Autodesk Fusion 360 part; units mm, degrees
(part 15 of 25)
  arc A3929 (0.7747, 17.3038) -> (0.7747, 16.9862) centre (0.7747, 17.145) ccw
  arc A3930 (40.64, 16.6688) -> (40.64, 16.3513) centre (40.64, 16.51) ccw
  arc A3931 (45.607, 16.3513) -> (45.607, 16.6688) centre (45.607, 16.51) ccw
  arc A3932 (16.0714, 16.6688) -> (16.0714, 16.3513) centre (16.0714, 16.51) ccw
  arc A3933 (44.7421, 18.8912) -> (44.7421, 19.2088) centre (44.7421, 19.05) ccw
  arc A3934 (53.34, 16.3513) -> (53.34, 16.6688) centre (53.34, 16.51) ccw
  arc A3935 (44.972, 16.9862) -> (44.972, 17.3038) centre (44.972, 17.145) ccw
  arc A3936 (68.404, 17.3038) -> (68.404, 16.9862) centre (68.404, 17.145) ccw
  arc A3937 (53.34, 17.9388) -> (53.34, 17.6212) centre (53.34, 17.78) ccw
  arc A3938 (49.2073, 16.9862) -> (49.2073, 17.3038) centre (49.2073, 17.145) ccw
  arc A3939 (24.1735, 17.6212) -> (24.1735, 17.9388) centre (24.1735, 17.78) ccw
  arc A3940 (26.7135, 17.6212) -> (26.7135, 17.9388) centre (26.7135, 17.78) ccw
  arc A3941 (29.2535, 17.6212) -> (29.2535, 17.9388) centre (29.2535, 17.78) ccw
  arc A3942 (57.898, 18.5738) -> (57.898, 18.2562) centre (57.898, 18.415) ccw
  arc A3943 (73.5304, 18.2562) -> (73.5304, 18.5738) centre (73.5304, 18.415) ccw
  arc A3944 (68.2336, 17.6212) -> (68.2336, 17.9388) centre (68.2336, 17.78) ccw
  arc A3945 (49.6453, 16.3513) -> (49.6453, 16.6688) centre (49.6453, 16.51) ccw
  arc A3946 (84.2253, 16.9862) -> (84.2253, 17.3038) centre (84.2253, 17.145) ccw
  arc A3947 (70.8314, 18.5738) -> (70.8314, 18.2562) centre (70.8314, 18.415) ccw
  arc A3948 (46.6979, 19.2088) -> (46.6979, 18.8912) centre (46.6979, 19.05) ccw
  arc A3949 (53.34, 16.6688) -> (53.34, 16.3513) centre (53.34, 16.51) ccw
  arc A3950 (54.7705, 17.3038) -> (54.7705, 16.9862) centre (54.7705, 17.145) ccw
  arc A3951 (34.2465, 17.9388) -> (34.2465, 17.6212) centre (34.2465, 17.78) ccw
  arc A3952 (40.64, 16.9862) -> (40.64, 17.3038) centre (40.64, 17.145) ccw
  arc A3953 (56.402, 16.9862) -> (56.402, 17.3038) centre (56.402, 17.145) ccw
  arc A3954 (54.1355, 16.6688) -> (54.1355, 16.3513) centre (54.1355, 16.51) ccw
  arc A3955 (24.0865, 17.9388) -> (24.0865, 17.6212) centre (24.0865, 17.78) ccw
  arc A3956 (40.64, 17.3038) -> (40.64, 16.9862) centre (40.64, 17.145) ccw
  arc A3957 (80.0328, 18.2562) -> (80.0328, 18.5738) centre (80.0328, 18.415) ccw
  arc A3958 (0.7747, 19.2088) -> (0.7747, 18.8912) centre (0.7747, 19.05) ccw
  arc A3959 (51.9547, 19.2088) -> (51.9547, 18.8912) centre (51.9547, 19.05) ccw
  arc A3960 (55.767, 17.6212) -> (55.767, 17.9388) centre (55.767, 17.78) ccw
  line L1372 (57.263, 19.05) -> (57.5886, 19.05)
  arc A3961 (81.5721, 18.2562) -> (81.5721, 18.5738) centre (81.5721, 18.415) ccw
  arc A3962 (36.7865, 17.9388) -> (36.7865, 17.6212) centre (36.7865, 17.78) ccw
  arc A3963 (54.1355, 19.2088) -> (54.1355, 18.8912) centre (54.1355, 19.05) ccw
  arc A3964 (0.7747, 18.5738) -> (0.7747, 18.2562) centre (0.7747, 18.415) ccw
  arc A3965 (40.64, 17.6212) -> (40.64, 17.9388) centre (40.64, 17.78) ccw
  arc A3966 (83.5279, 19.8438) -> (83.5279, 19.5263) centre (83.5279, 19.6851) ccw
  arc A3967 (84.2253, 19.5263) -> (84.2253, 19.8438) centre (84.2253, 19.6851) ccw
  arc A3968 (40.64, 17.9388) -> (40.64, 17.6212) centre (40.64, 17.78) ccw
  line L1373 (39.3265, 17.78) -> (39.8168, 17.78)
  arc A3969 (56.9341, 20.1612) -> (56.9341, 20.4788) centre (56.9341, 20.32) ccw
  arc A3970 (70.1964, 20.4788) -> (70.1964, 20.1612) centre (70.1964, 20.32) ccw
  arc A3971 (44.7421, 20.1612) -> (44.7421, 20.4788) centre (44.7421, 20.32) ccw
  arc A3972 (6.2857, 20.1612) -> (6.2857, 20.4788) centre (6.2857, 20.32) ccw
  arc A3973 (36.8735, 17.6212) -> (36.8735, 17.9388) centre (36.8735, 17.78) ccw
  arc A3974 (83.5279, 18.5738) -> (83.5279, 18.2562) centre (83.5279, 18.415) ccw
  arc A3975 (44.7421, 18.2562) -> (44.7421, 18.5738) centre (44.7421, 18.415) ccw
  arc A3976 (41.4632, 17.9388) -> (41.4632, 17.6212) centre (41.4632, 17.78) ccw
  arc A3977 (79.2208, 20.1612) -> (79.2208, 20.4788) centre (79.2208, 20.32) ccw
  line L1374 (81.4096, 18.415) -> (81.5721, 18.415)
  arc A3978 (53.34, 18.5738) -> (53.34, 18.2562) centre (53.34, 18.415) ccw
  arc A3979 (72.7184, 20.1612) -> (72.7184, 20.4788) centre (72.7184, 20.32) ccw
  arc A3980 (84.2253, 20.1612) -> (84.2253, 20.4788) centre (84.2253, 20.32) ccw
  arc A3981 (8.9543, 20.4788) -> (8.9543, 20.1612) centre (8.9543, 20.32) ccw
  arc A3982 (46.6979, 18.5738) -> (46.6979, 18.2562) centre (46.6979, 18.415) ccw
  arc A3983 (75.7192, 20.4788) -> (75.7192, 20.1612) centre (75.7192, 20.32) ccw
  arc A3984 (59.2514, 19.2088) -> (59.2514, 18.8912) centre (59.2514, 19.05) ccw
  arc A3985 (83.3742, 20.4788) -> (83.3742, 20.1612) centre (83.3742, 20.32) ccw
  line L1375 (36.7865, 17.78) -> (36.8735, 17.78)
  arc A3986 (7.62, 20.1612) -> (7.62, 20.4788) centre (7.62, 20.32) ccw
  arc A3987 (39.8168, 17.6212) -> (39.8168, 17.9388) centre (39.8168, 17.78) ccw
  line L1376 (54.7705, 18.415) -> (55.132, 18.415)
  arc A3988 (53.34, 18.2562) -> (53.34, 18.5738) centre (53.34, 18.415) ccw
  arc A3989 (81.4096, 18.5738) -> (81.4096, 18.2562) centre (81.4096, 18.415) ccw
  arc A3990 (74.9072, 18.5738) -> (74.9072, 18.2562) centre (74.9072, 18.415) ccw
  arc A3991 (53.34, 19.2088) -> (53.34, 18.8912) centre (53.34, 19.05) ccw
  arc A3992 (44.7421, 17.6212) -> (44.7421, 17.9388) centre (44.7421, 17.78) ccw
  arc A3993 (47.103, 17.9388) -> (47.103, 17.6212) centre (47.103, 17.78) ccw
  arc A3994 (84.2253, 17.6212) -> (84.2253, 17.9388) centre (84.2253, 17.78) ccw
  arc A3995 (49.2073, 18.2562) -> (49.2073, 18.5738) centre (49.2073, 18.415) ccw
  arc A3996 (53.34, 18.8912) -> (53.34, 19.2088) centre (53.34, 19.05) ccw
  arc A3997 (49.0855, 17.6212) -> (49.0855, 17.9388) centre (49.0855, 17.78) ccw
  arc A3998 (54.9021, 18.8912) -> (54.9021, 19.2088) centre (54.9021, 19.05) ccw
  arc A3999 (58.533, 17.9388) -> (58.533, 17.6212) centre (58.533, 17.78) ccw
  arc A4000 (55.132, 18.2562) -> (55.132, 18.5738) centre (55.132, 18.415) ccw
  arc A4001 (67.6058, 18.2562) -> (67.6058, 18.5738) centre (67.6058, 18.415) ccw
  arc A4002 (84.2253, 18.2562) -> (84.2253, 18.5738) centre (84.2253, 18.415) ccw
  arc A4003 (0.7747, 21.1138) -> (0.7747, 20.7963) centre (0.7747, 20.955) ccw
  arc A4004 (7.62, 21.1138) -> (7.62, 20.7963) centre (7.62, 20.955) ccw
  arc A4005 (56.9536, 19.5263) -> (56.9536, 19.8438) centre (56.9536, 19.6851) ccw
  arc A4006 (7.62, 20.4788) -> (7.62, 20.1612) centre (7.62, 20.32) ccw
  arc A4007 (57.5886, 18.8912) -> (57.5886, 19.2088) centre (57.5886, 19.05) ccw
  arc A4008 (57.263, 19.2088) -> (57.263, 18.8912) centre (57.263, 19.05) ccw
  arc A4009 (83.5279, 19.2088) -> (83.5279, 18.8912) centre (83.5279, 19.05) ccw
  arc A4010 (5.7785, 20.7963) -> (5.7785, 21.1138) centre (5.7785, 20.955) ccw
  arc A4011 (7.62, 20.7963) -> (7.62, 21.1138) centre (7.62, 20.955) ccw
  arc A4012 (84.2253, 18.8912) -> (84.2253, 19.2088) centre (84.2253, 19.05) ccw
  arc A4013 (74.9072, 19.8438) -> (74.9072, 19.5263) centre (74.9072, 19.6851) ccw
  arc A4014 (0.7747, 19.8438) -> (0.7747, 19.5263) centre (0.7747, 19.6851) ccw
  arc A4015 (46.6979, 20.4788) -> (46.6979, 20.1612) centre (46.6979, 20.32) ccw
  line L1377 (56.8579, 20.32) -> (56.9341, 20.32)
  arc A4016 (56.8579, 20.4788) -> (56.8579, 20.1612) centre (56.8579, 20.32) ccw
  arc A4017 (67.0941, 20.1612) -> (67.0941, 20.4788) centre (67.0941, 20.32) ccw
  arc A4018 (59.9059, 20.4788) -> (59.9059, 20.1612) centre (59.9059, 20.32) ccw
  arc A4019 (0.7747, 20.4788) -> (0.7747, 20.1612) centre (0.7747, 20.32) ccw
  arc A4020 (46.6979, 19.8438) -> (46.6979, 19.5263) centre (46.6979, 19.6851) ccw
  arc A4021 (54.9021, 19.5263) -> (54.9021, 19.8438) centre (54.9021, 19.6851) ccw
  arc A4022 (71.4591, 21.7488) -> (71.4591, 21.4312) centre (71.4591, 21.59) ccw
  arc A4023 (84.2253, 21.4312) -> (84.2253, 21.7488) centre (84.2253, 21.59) ccw
  arc A4024 (44.7421, 19.5263) -> (44.7421, 19.8438) centre (44.7421, 19.6851) ccw
  arc A4025 (81.5721, 18.8912) -> (81.5721, 19.2088) centre (81.5721, 19.05) ccw
  arc A4026 (7.62, 22.0663) -> (7.62, 22.3838) centre (7.62, 22.2251) ccw
  arc A4027 (7.62, 22.3838) -> (7.62, 22.0663) centre (7.62, 22.2251) ccw
  arc A4028 (56.8579, 21.7488) -> (56.8579, 21.4312) centre (56.8579, 21.59) ccw
  line L1378 (56.8579, 19.685) -> (56.9536, 19.685)
  line L1379 (56.8579, 20.955) -> (56.9536, 20.955)
  arc A4029 (56.8579, 19.8438) -> (56.8579, 19.5263) centre (56.8579, 19.6851) ccw
  arc A4030 (44.464, 20.7963) -> (44.464, 21.1138) centre (44.464, 20.955) ccw
  arc A4031 (43.194, 22.0663) -> (43.194, 22.3838) centre (43.194, 22.2251) ccw
  arc A4032 (70.0464, 19.8438) -> (70.0464, 19.5263) centre (70.0464, 19.6851) ccw
  arc A4033 (70.1964, 19.2088) -> (70.1964, 18.8912) centre (70.1964, 19.05) ccw
  arc A4034 (67.437, 18.8912) -> (67.437, 19.2088) centre (67.437, 19.05) ccw
  arc A4035 (54.9021, 20.1612) -> (54.9021, 20.4788) centre (54.9021, 20.32) ccw
  arc A4036 (59.8864, 19.8438) -> (59.8864, 19.5263) centre (59.8864, 19.6851) ccw
  arc A4037 (80.0328, 19.5263) -> (80.0328, 19.8438) centre (80.0328, 19.6851) ccw
  arc A4038 (59.2514, 21.7488) -> (59.2514, 21.4312) centre (59.2514, 21.59) ccw
  arc A4039 (73.5304, 19.5263) -> (73.5304, 19.8438) centre (73.5304, 19.6851) ccw
  arc A4040 (72.4535, 21.4312) -> (72.4535, 21.7488) centre (72.4535, 21.59) ccw
  arc A4041 (67.1136, 19.5263) -> (67.1136, 19.8438) centre (67.1136, 19.6851) ccw
  arc A4042 (5.7785, 22.0663) -> (5.7785, 22.3838) centre (5.7785, 22.2251) ccw
  arc A4043 (48.9268, 17.439) -> (49.2443, 17.439) centre (49.0856, 17.439) ccw
  line L1380 (53.34, 17.78) -> (53.34, 16.3195)
  line L1381 (51.7712, 16.3265) -> (52.2496, 16.8049)
  arc A4044 (54.6417, 17.175) -> (54.9592, 17.175) centre (54.8005, 17.175) ccw
  arc A4045 (57.5886, 21.4312) -> (57.5886, 21.7488) centre (57.5886, 21.59) ccw
  arc A4046 (82.7392, 21.1138) -> (82.7392, 20.7963) centre (82.7392, 20.955) ccw
  arc A4047 (53.1813, 17.78) -> (53.4988, 17.78) centre (53.3401, 17.78) ccw
  arc A4048 (45.96, 22.3838) -> (45.96, 22.0663) centre (45.96, 22.2251) ccw
  arc A4049 (54.9021, 22.0663) -> (54.9021, 22.3838) centre (54.9021, 22.2251) ccw
  arc A4050 (53.34, 17.9387) -> (53.34, 17.6212) centre (53.34, 17.78) ccw
  arc A4051 (54.9021, 20.7963) -> (54.9021, 21.1138) centre (54.9021, 20.955) ccw
  arc A4052 (48.9388, 18.1818) -> (49.2322, 18.0603) centre (49.0855, 18.1211) ccw
  line L1382 (54.8005, 17.175) -> (54.8005, 17.78)
  arc A4053 (53.4987, 17.78) -> (53.1812, 17.78) centre (53.34, 17.78) ccw
  arc A4054 (56.8579, 21.1138) -> (56.8579, 20.7963) centre (56.8579, 20.955) ccw
  arc A4055 (72.4553, 20.7963) -> (72.4553, 21.1138) centre (72.4553, 20.955) ccw
  arc A4056 (54.9592, 18.385) -> (54.6417, 18.385) centre (54.8005, 18.385) ccw
  line L1383 (54.8005, 18.385) -> (53.945, 19.2405)
  line L1384 (49.8288, 19.2335) -> (49.3465, 18.7512)
  arc A4057 (0.7747, 22.3838) -> (0.7747, 22.0663) centre (0.7747, 22.2251) ccw
  line L1385 (54.8005, 17.78) -> (53.34, 17.78)
  line L1386 (54.8005, 17.78) -> (54.8005, 18.385)
  arc A4058 (51.6589, 16.4388) -> (51.8834, 16.2143) centre (51.7712, 16.3266) ccw
  line L1387 (53.34, 16.3195) -> (53.945, 16.3195)
  arc A4059 (46.6979, 21.1138) -> (46.6979, 20.7963) centre (46.6979, 20.955) ccw
  arc A4060 (53.1813, 16.3195) -> (53.4988, 16.3195) centre (53.3401, 16.3195) ccw
  arc A4061 (51.141, 15.9068) -> (51.141, 16.2243) centre (51.141, 16.0655) ccw
  line L1388 (52.2496, 16.8049) -> (52.735, 16.3195)
  arc A4062 (53.945, 16.1608) -> (53.945, 16.4783) centre (53.945, 16.3195) ccw
  arc A4063 (82.663, 21.7488) -> (82.663, 21.4312) centre (82.663, 21.59) ccw
  arc A4064 (7.62, 21.7488) -> (7.62, 21.4312) centre (7.62, 21.59) ccw
  arc A4065 (54.9021, 21.4312) -> (54.9021, 21.7488) centre (54.9021, 21.59) ccw
  arc A4066 (67.1136, 20.7963) -> (67.1136, 21.1138) centre (67.1136, 20.955) ccw
  arc A4067 (56.9536, 20.7963) -> (56.9536, 21.1138) centre (56.9536, 20.955) ccw
  arc A4068 (54.0572, 19.3528) -> (53.8327, 19.1282) centre (53.945, 19.2405) ccw
  arc A4069 (70.8314, 21.1138) -> (70.8314, 20.7963) centre (70.8314, 20.955) ccw
  line L1389 (53.945, 19.2405) -> (53.34, 19.2405)
  arc A4070 (67.7486, 21.4312) -> (67.7486, 21.7488) centre (67.7486, 21.59) ccw
  arc A4071 (52.6228, 16.2072) -> (52.8473, 16.4318) centre (52.7351, 16.3195) ccw
  arc A4072 (54.8005, 17.6213) -> (54.8005, 17.9388) centre (54.8005, 17.78) ccw
  arc A4073 (9.4615, 22.3838) -> (9.4615, 22.0663) centre (9.4615, 22.2251) ccw
  line L1390 (53.34, 17.78) -> (54.8005, 17.78)
  arc A4074 (46.3862, 22.0233) -> (46.1617, 21.7988) centre (46.2739, 21.9111) ccw
  arc A4075 (84.2253, 20.7963) -> (84.2253, 21.1138) centre (84.2253, 20.955) ccw
  arc A4076 (9.4615, 21.1138) -> (9.4615, 20.7963) centre (9.4615, 20.955) ccw
  arc A4077 (0.7747, 21.7488) -> (0.7747, 21.4312) centre (0.7747, 21.59) ccw
  arc A4078 (43.829, 21.4312) -> (43.829, 21.7488) centre (43.829, 21.59) ccw
  arc A4079 (46.568, 21.7488) -> (46.568, 21.4312) centre (46.568, 21.59) ccw
  arc A4080 (49.4932, 18.6904) -> (49.1998, 18.8119) centre (49.3465, 18.7512) ccw
  arc A4081 (53.34, 17.9388) -> (53.34, 17.6213) centre (53.34, 17.78) ccw
  line L1391 (46.2739, 21.911) -> (43.1258, 25.0591)
  arc A4082 (7.62, 21.4312) -> (7.62, 21.7488) centre (7.62, 21.59) ccw
  arc A4083 (59.8864, 21.1138) -> (59.8864, 20.7963) centre (59.8864, 20.955) ccw
  arc A4084 (54.6417, 17.78) -> (54.9592, 17.78) centre (54.8005, 17.78) ccw
  arc A4085 (12.1476, 33.5781) -> (12.465, 33.5781) centre (12.3063, 33.5781) ccw
  line L1392 (51.141, 16.0655) -> (51.7712, 16.3265)
  arc A4086 (49.1998, 16.7481) -> (49.4932, 16.8696) centre (49.3465, 16.8088) ccw
  arc A4087 (49.9411, 19.1212) -> (49.7166, 19.3457) centre (49.8288, 19.2335) ccw
  line L1393 (49.3465, 16.8088) -> (49.8288, 16.3265)
  arc A4088 (52.3619, 16.9172) -> (52.1374, 16.6927) centre (52.2497, 16.8049) ccw
  line L1394 (53.945, 16.3195) -> (54.8005, 17.175)
  arc A4089 (53.34, 16.4783) -> (53.34, 16.1608) centre (53.34, 16.3195) ccw
  arc A4090 (51.0803, 16.2122) -> (51.2018, 15.9188) centre (51.1411, 16.0655) ccw
  arc A4091 (50.459, 16.2243) -> (50.459, 15.9068) centre (50.459, 16.0655) ccw
  arc A4092 (53.8327, 16.4318) -> (54.0572, 16.2072) centre (53.9449, 16.3195) ccw
  arc A4093 (54.9592, 17.78) -> (54.6417, 17.78) centre (54.8005, 17.78) ccw
  arc A4094 (54.9128, 17.0628) -> (54.6882, 17.2873) centre (54.8005, 17.175) ccw
  arc A4095 (49.2443, 18.121) -> (48.9268, 18.121) centre (49.0856, 18.121) ccw
  arc A4096 (49.2343, 18.8634) -> (49.4588, 18.6389) centre (49.3465, 18.7512) ccw
  arc A4097 (53.34, 16.1608) -> (53.34, 16.4783) centre (53.34, 16.3195) ccw
  arc A4098 (52.3619, 16.6927) -> (52.1374, 16.9172) centre (52.2497, 16.805) ccw
  line L1395 (49.3465, 18.7512) -> (49.0855, 18.121)
  arc A4099 (53.34, 17.9387) -> (53.34, 17.6212) centre (53.34, 17.78) ccw
  line L1396 (52.735, 16.3195) -> (53.34, 16.3195)
  arc A4100 (49.8896, 16.4732) -> (49.7681, 16.1798) centre (49.8289, 16.3265) ccw
  arc A4101 (53.1812, 16.3195) -> (53.4987, 16.3195) centre (53.34, 16.3195) ccw
  arc A4102 (51.8319, 16.1798) -> (51.7104, 16.4732) centre (51.7712, 16.3265) ccw
  arc A4103 (53.4988, 17.78) -> (53.1813, 17.78) centre (53.3401, 17.78) ccw
  line L1397 (53.34, 16.3195) -> (53.34, 17.78)
  line L1398 (49.8288, 16.3265) -> (50.459, 16.0655)
  line L1399 (50.459, 16.0655) -> (51.141, 16.0655)
  line L1400 (49.0855, 17.439) -> (49.3465, 16.8088)
  arc A4104 (52.735, 16.4783) -> (52.735, 16.1608) centre (52.735, 16.3195) ccw
  line L1401 (49.0855, 18.121) -> (49.0855, 17.439)
  arc A4105 (50.3982, 15.9188) -> (50.5197, 16.2122) centre (50.459, 16.0655) ccw
  arc A4106 (54.8005, 17.6212) -> (54.8005, 17.9387) centre (54.8005, 17.78) ccw
  arc A4107 (53.34, 17.6212) -> (53.34, 17.9387) centre (53.34, 17.78) ccw
  arc A4108 (49.7166, 16.2143) -> (49.9411, 16.4388) centre (49.8288, 16.3266) ccw
  arc A4109 (49.2322, 17.4997) -> (48.9388, 17.3782) centre (49.0855, 17.439) ccw
  arc A4110 (49.4588, 16.9211) -> (49.2343, 16.6966) centre (49.3465, 16.8089) ccw
  arc A4111 (53.4988, 17.78) -> (53.1813, 17.78) centre (53.3401, 17.78) ccw
  arc A4112 (73.8187, 45.72) -> (73.5012, 45.72) centre (73.66, 45.72) ccw
  line L1402 (49.53, 40.64) -> (50.8, 41.91)
  arc A4113 (13.8113, 33.909) -> (14.1288, 33.909) centre (13.9701, 33.909) ccw
  arc A4114 (21.59, 12.5413) -> (21.59, 12.8588) centre (21.59, 12.7001) ccw
  line L1403 (33.02, 6.35) -> (35.56, 6.35)
  arc A4115 (15.1531, 11.5296) -> (15.3777, 11.305) centre (15.2654, 11.4173) ccw
  arc A4116 (72.5023, 47.1023) -> (72.2777, 46.8777) centre (72.39, 46.99) ccw
  arc A4117 (35.56, 6.1913) -> (35.56, 6.5088) centre (35.56, 6.3501) ccw
  arc A4118 (80.7491, 2.7242) -> (80.7491, 3.0417) centre (80.7491, 2.883) ccw
  arc A4119 (73.8187, 44.45) -> (73.5012, 44.45) centre (73.66, 44.45) ccw
  line L1404 (80.7212, 16.7894) -> (74.2188, 16.7894)
  arc A4120 (16.5481, 12.8588) -> (16.5481, 12.5413) centre (16.5481, 12.7001) ccw
  arc A4121 (3.1603, 40.2443) -> (2.9357, 40.0197) centre (3.048, 40.132) ccw
  line L1405 (80.7491, 2.8829) -> (74.2467, 2.8829)
  line L1406 (21.59, 12.7) -> (22.86, 13.97)
  arc A4122 (13.8577, 35.4477) -> (14.0823, 35.6723) centre (13.97, 35.56) ccw
  line L1407 (3.048, 41.91) -> (3.048, 40.132)
  arc A4123 (14.1288, 35.56) -> (13.8113, 35.56) centre (13.9701, 35.56) ccw
  arc A4124 (72.2313, 46.99) -> (72.5487, 46.99) centre (72.39, 46.99) ccw
  arc A4125 (80.7212, 16.6306) -> (80.7212, 16.9482) centre (80.7212, 16.7894) ccw
  line L1408 (50.8, 41.91) -> (52.07, 43.18)
  arc A4126 (11.43, 37.9413) -> (11.43, 38.2587) centre (11.43, 38.1) ccw
  arc A4127 (43.2923, 40.5277) -> (43.0677, 40.7523) centre (43.18, 40.64) ccw
  arc A4128 (50.6877, 42.0223) -> (50.9123, 41.7977) centre (50.8, 41.91) ccw
  line L1409 (13.97, 35.56) -> (13.97, 33.909)
  arc A4129 (33.02, 6.5088) -> (33.02, 6.1913) centre (33.02, 6.3501) ccw
  arc A4130 (73.5477, 45.6077) -> (73.7723, 45.8323) centre (73.66, 45.72) ccw
  line L1410 (3.048, 40.132) -> (5.08, 38.1)
  arc A4131 (74.2467, 3.0417) -> (74.2467, 2.7242) centre (74.2467, 2.883) ccw
  line L1411 (52.07, 43.18) -> (58.42, 43.18)
  line L1412 (43.18, 40.64) -> (49.53, 40.64)
  arc A4132 (21.4777, 12.8123) -> (21.7023, 12.5877) centre (21.59, 12.7) ccw
  arc A4133 (74.2188, 16.6306) -> (74.2188, 16.9482) centre (74.2188, 16.7894) ccw
  arc A4134 (50.6877, 29.0977) -> (50.9123, 29.3223) centre (50.8, 29.21) ccw
  arc A4135 (5.08, 38.2587) -> (5.08, 37.9413) centre (5.08, 38.1) ccw
  line L1413 (16.5481, 12.7) -> (21.59, 12.7)
  arc A4136 (73.5012, 31.75) -> (73.8187, 31.75) centre (73.66, 31.75) ccw
  arc A4137 (74.2188, 16.9482) -> (74.2188, 16.6306) centre (74.2188, 16.7894) ccw
  arc A4138 (2.8893, 40.132) -> (3.2067, 40.132) centre (3.048, 40.132) ccw
  line L1414 (73.66, 45.72) -> (72.39, 46.99)
  arc A4139 (68.4213, 19.05) -> (68.7387, 19.05) centre (68.58, 19.05) ccw
  arc A4140 (16.6604, 12.5877) -> (16.4358, 12.8123) centre (16.5481, 12.7) ccw
  arc A4141 (50.9588, 29.21) -> (50.6413, 29.21) centre (50.8001, 29.21) ccw
  line L1415 (15.2654, 11.4173) -> (16.5481, 12.7)
  arc A4142 (3.2067, 41.91) -> (2.8893, 41.91) centre (3.048, 41.91) ccw
  arc A4143 (49.53, 40.4813) -> (49.53, 40.7987) centre (49.53, 40.64) ccw
  arc A4144 (40.5277, 38.2123) -> (40.7523, 37.9877) centre (40.64, 38.1) ccw
  line L1416 (22.86, 13.97) -> (22.86, 16.51)
  arc A4145 (43.18, 40.7987) -> (43.18, 40.4813) centre (43.18, 40.64) ccw
  arc A4146 (22.7012, 13.97) -> (23.0188, 13.97) centre (22.86, 13.97) ccw
  line L1417 (40.64, 33.02) -> (46.99, 33.02)
  arc A4147 (47.1023, 33.1323) -> (46.8777, 32.9077) centre (46.99, 33.02) ccw
  line L1418 (73.66, 44.45) -> (73.66, 45.72)
  line L1419 (5.08, 38.1) -> (11.43, 38.1)
  line L1420 (73.66, 31.75) -> (73.66, 44.45)
  arc A4148 (11.5423, 38.2123) -> (11.3177, 37.9877) centre (11.43, 38.1) ccw
  line L1421 (11.43, 38.1) -> (13.97, 35.56)
  line L1422 (72.39, 46.99) -> (72.39, 49.53)
  arc A4149 (4.9677, 37.9877) -> (5.1923, 38.2123) centre (5.08, 38.1) ccw
  arc A4150 (23.0188, 16.51) -> (22.7012, 16.51) centre (22.86, 16.51) ccw
  arc A4151 (22.9723, 13.8577) -> (22.7477, 14.0823) centre (22.86, 13.97) ccw
  arc A4152 (73.5012, 44.45) -> (73.8187, 44.45) centre (73.66, 44.45) ccw
  arc A4153 (72.5487, 49.53) -> (72.2313, 49.53) centre (72.39, 49.53) ccw
  arc A4154 (16.002, 26.0668) -> (16.002, 25.7492) centre (16.002, 25.908) ccw
  arc A4155 (73.5012, 29.21) -> (73.8187, 29.21) centre (73.66, 29.21) ccw
  line L1423 (63.5, 31.75) -> (63.5, 29.21)
  arc A4156 (40.64, 33.1788) -> (40.64, 32.8613) centre (40.64, 33.0201) ccw
  line L1424 (68.58, 20.32) -> (70.485, 22.225)
  arc A4157 (26.5113, 25.4) -> (26.8288, 25.4) centre (26.67, 25.4) ccw
  line L1425 (68.58, 19.05) -> (68.58, 20.32)
  line L1426 (26.67, 29.21) -> (26.67, 25.4)
  arc A4158 (58.42, 43.0213) -> (58.42, 43.3387) centre (58.42, 43.18) ccw
  line L1427 (46.99, 33.02) -> (50.8, 29.21)
  line L1428 (33.02, 6.35) -> (30.48, 6.35)
  arc A4159 (26.67, 25.2413) -> (26.67, 25.5588) centre (26.67, 25.4001) ccw
  arc A4160 (73.7723, 29.0977) -> (73.5477, 29.3223) centre (73.66, 29.21) ccw
  line L1429 (73.66, 29.21) -> (73.66, 31.75)
  line L1430 (50.8, 29.21) -> (50.8, 25.4)
  arc A4161 (30.3677, 6.2377) -> (30.5923, 6.4623) centre (30.48, 6.35) ccw
  arc A4162 (46.99, 32.8613) -> (46.99, 33.1788) centre (46.99, 33.0201) ccw
  line L1431 (72.39, 27.94) -> (70.485, 27.94)
  arc A4163 (68.4677, 20.4323) -> (68.6923, 20.2077) centre (68.58, 20.32) ccw
  line L1432 (73.66, 29.21) -> (72.39, 27.94)
  arc A4164 (21.59, 25.5588) -> (21.59, 25.2413) centre (21.59, 25.4001) ccw
  arc A4165 (52.07, 43.3387) -> (52.07, 43.0213) centre (52.07, 43.18) ccw
  arc A4166 (49.4177, 40.7523) -> (49.6423, 40.5277) centre (49.53, 40.64) ccw
  arc A4167 (21.1943, 26.0203) -> (20.9697, 25.7957) centre (21.082, 25.908) ccw
  arc A4168 (70.8406, 16.9482) -> (70.8406, 16.6306) centre (70.8406, 16.7894) ccw
  arc A4169 (37.9877, 30.5923) -> (38.2123, 30.3677) centre (38.1, 30.48) ccw
  arc A4170 (22.9723, 14.0823) -> (22.7477, 13.8577) centre (22.86, 13.97) ccw
  arc A4171 (21.4777, 25.2877) -> (21.7023, 25.5123) centre (21.59, 25.4) ccw
  arc A4172 (50.6413, 25.4) -> (50.9588, 25.4) centre (50.8001, 25.4) ccw
  line L1433 (16.002, 25.908) -> (21.082, 25.908)
  arc A4173 (63.6587, 31.75) -> (63.3413, 31.75) centre (63.5, 31.75) ccw
  arc A4174 (70.7283, 16.6771) -> (70.9529, 16.9017) centre (70.8406, 16.7894) ccw
  line L1434 (70.485, 22.225) -> (70.485, 27.94)
  line L1435 (40.64, 33.02) -> (38.1, 30.48)
  arc A4175 (63.3413, 29.21) -> (63.6587, 29.21) centre (63.5, 29.21) ccw
  arc A4176 (33.02, 6.1913) -> (33.02, 6.5088) centre (33.02, 6.3501) ccw
  arc A4177 (64.77, 28.0988) -> (64.77, 27.7813) centre (64.77, 27.9401) ccw
  arc A4178 (70.485, 28.0988) -> (70.485, 27.7813) centre (70.485, 27.9401) ccw
  arc A4179 (68.7387, 20.32) -> (68.4213, 20.32) centre (68.58, 20.32) ccw
  arc A4180 (70.3263, 22.225) -> (70.6437, 22.225) centre (70.485, 22.225) ccw
  arc A4181 (70.5973, 22.1127) -> (70.3727, 22.3373) centre (70.485, 22.225) ccw
  arc A4182 (26.5577, 29.3223) -> (26.7823, 29.0977) centre (26.67, 29.21) ccw
  arc A4183 (21.082, 25.7492) -> (21.082, 26.0668) centre (21.082, 25.908) ccw
  line L1436 (74.2188, 16.7894) -> (70.8406, 16.7894)
  arc A4184 (28.0523, 30.3677) -> (27.8277, 30.5923) centre (27.94, 30.48) ccw
  arc A4185 (70.6437, 27.94) -> (70.3263, 27.94) centre (70.485, 27.94) ccw
  arc A4186 (73.8187, 31.75) -> (73.5012, 31.75) centre (73.66, 31.75) ccw
  line L1437 (70.8406, 16.7894) -> (68.58, 19.05)
  arc A4187 (50.9123, 41.7977) -> (50.6877, 42.0223) centre (50.8, 41.91) ccw
  arc A4188 (27.94, 30.6388) -> (27.94, 30.3212) centre (27.94, 30.48) ccw
  line L1438 (30.48, 6.35) -> (22.86, 13.97)
  line L1439 (64.77, 27.94) -> (70.485, 27.94)
  arc A4189 (30.48, 6.5088) -> (30.48, 6.1913) centre (30.48, 6.3501) ccw
  arc A4190 (72.2777, 28.0523) -> (72.5023, 27.8277) centre (72.39, 27.94) ccw
  line L1440 (21.59, 25.4) -> (26.67, 25.4)
  arc A4191 (40.7523, 32.9077) -> (40.5277, 33.1323) centre (40.64, 33.02) ccw
  arc A4192 (52.1823, 43.0677) -> (51.9577, 43.2923) centre (52.07, 43.18) ccw
  line L1441 (21.082, 25.908) -> (21.59, 25.4)
  line L1442 (38.1, 30.48) -> (27.94, 30.48)
  line L1443 (40.64, 38.1) -> (43.18, 40.64)
  line L1444 (63.5, 29.21) -> (64.77, 27.94)
  arc A4193 (68.6923, 19.1623) -> (68.4677, 18.9377) centre (68.58, 19.05) ccw
  arc A4194 (71.12, 39.2938) -> (71.12, 39.4462) centre (71.12, 39.37) ccw
  arc A4195 (52.1239, 39.3161) -> (52.0161, 39.4239) centre (52.07, 39.37) ccw
  arc A4196 (16.8402, 44.196) -> (16.6878, 44.196) centre (16.764, 44.196) ccw
  line L1445 (13.081, 30.48) -> (9.271, 34.29)
  arc A4197 (3.048, 34.3662) -> (3.048, 34.2138) centre (3.048, 34.29) ccw
  line L1446 (78.74, 31.75) -> (78.74, 44.45)
  arc A4198 (14.0239, 47.0439) -> (13.9161, 46.9361) centre (13.97, 46.99) ccw
  arc A4199 (8.128, 34.2138) -> (8.128, 34.3662) centre (8.128, 34.29) ccw
  arc A4200 (13.8938, 46.99) -> (14.0462, 46.99) centre (13.97, 46.99) ccw
  line L1447 (54.61, 36.83) -> (71.12, 36.83)
  arc A4201 (45.7962, 13.97) -> (45.6438, 13.97) centre (45.72, 13.97) ccw
  arc A4202 (50.7461, 33.0739) -> (50.8539, 32.9661) centre (50.8, 33.02) ccw
  line L1448 (52.07, 39.37) -> (71.12, 39.37)
  arc A4203 (76.1238, 31.75) -> (76.2762, 31.75) centre (76.2, 31.75) ccw
  arc A4204 (64.6577, 27.8277) -> (64.8823, 28.0523) centre (64.77, 27.94) ccw
  arc A4205 (52.07, 39.4462) -> (52.07, 39.2938) centre (52.07, 39.37) ccw
  arc A4206 (54.61, 36.9062) -> (54.61, 36.7538) centre (54.61, 36.83) ccw
  arc A4207 (72.39, 27.7813) -> (72.39, 28.0988) centre (72.39, 27.9401) ccw
  line L1449 (50.8, 33.02) -> (54.61, 36.83)
  arc A4208 (14.0462, 49.53) -> (13.8938, 49.53) centre (13.97, 49.53) ccw
  line L1450 (45.72, 13.97) -> (45.72, 6.35)
  line L1451 (16.764, 44.196) -> (16.764, 32.004)
  arc A4209 (54.6639, 36.7761) -> (54.5561, 36.8839) centre (54.61, 36.83) ccw
  arc A4210 (78.6638, 31.75) -> (78.8162, 31.75) centre (78.74, 31.75) ccw
  line L1452 (16.764, 32.004) -> (15.24, 30.48)
  arc A4211 (16.6878, 32.004) -> (16.8402, 32.004) centre (16.764, 32.004) ccw
  arc A4212 (13.0271, 30.4261) -> (13.1349, 30.5339) centre (13.081, 30.48) ccw
  arc A4213 (8.128, 34.3662) -> (8.128, 34.2138) centre (8.128, 34.29) ccw
  arc A4214 (11.3538, 45.72) -> (11.5062, 45.72) centre (11.43, 45.72) ccw
  line L1453 (27.94, 30.48) -> (26.67, 29.21)
  arc A4215 (78.8162, 44.45) -> (78.6638, 44.45) centre (78.74, 44.45) ccw
  arc A4216 (63.6123, 29.3223) -> (63.3877, 29.0977) centre (63.5, 29.21) ccw
  arc A4217 (70.485, 27.7813) -> (70.485, 28.0988) centre (70.485, 27.9401) ccw
  arc A4218 (16.7101, 44.1421) -> (16.8179, 44.2499) centre (16.764, 44.196) ccw
  arc A4219 (74.2467, 7.4803) -> (74.2467, 7.3279) centre (74.2467, 7.4041) ccw
  line L1454 (80.7491, 7.4041) -> (82.677, 9.332)
  line L1455 (13.97, 46.99) -> (16.764, 44.196)
  arc A4220 (10.1061, 44.5039) -> (10.2139, 44.3961) centre (10.16, 44.45) ccw
  arc A4221 (76.2762, 44.45) -> (76.1238, 44.45) centre (76.2, 44.45) ccw
  arc A4222 (55.8038, 19.05) -> (55.9562, 19.05) centre (55.88, 19.05) ccw
  arc A4223 (13.081, 30.5562) -> (13.081, 30.4038) centre (13.081, 30.48) ccw
  arc A4224 (55.9339, 19.1039) -> (55.8261, 18.9961) centre (55.88, 19.05) ccw
  arc A4225 (80.6953, 7.458) -> (80.803, 7.3502) centre (80.7492, 7.4041) ccw
  arc A4226 (38.1, 30.3212) -> (38.1, 30.6388) centre (38.1, 30.48) ccw
  arc A4227 (50.7461, 38.1539) -> (50.8539, 38.0461) centre (50.8, 38.1) ccw
  line L1456 (3.048, 34.29) -> (8.128, 34.29)
  line L1457 (50.8, 38.1) -> (52.07, 39.37)
  arc A4228 (9.271, 34.2138) -> (9.271, 34.3662) centre (9.271, 34.29) ccw
  arc A4229 (26.8288, 29.21) -> (26.5113, 29.21) centre (26.67, 29.21) ccw
  arc A4230 (45.6438, 6.35) -> (45.7962, 6.35) centre (45.72, 6.35) ccw
  line L1458 (9.271, 34.29) -> (8.128, 34.29)
  line L1459 (76.2, 31.75) -> (76.2, 44.45)
  arc A4231 (16.8179, 31.9501) -> (16.7101, 32.0579) centre (16.764, 32.004) ccw
  arc A4232 (71.12, 36.7538) -> (71.12, 36.9062) centre (71.12, 36.83) ccw
  line L1460 (15.24, 30.48) -> (13.081, 30.48)
  arc A4233 (15.1861, 30.5339) -> (15.2939, 30.4261) centre (15.24, 30.48) ccw
  arc A4234 (15.24, 30.4038) -> (15.24, 30.5562) centre (15.24, 30.48) ccw
  line L1461 (13.97, 49.53) -> (13.97, 46.99)
  arc A4235 (9.3249, 34.3439) -> (9.2171, 34.2361) centre (9.271, 34.29) ccw
  line L1462 (71.7067, 7.4041) -> (68.9508, 10.16)
  arc A4236 (11.5062, 49.53) -> (11.3538, 49.53) centre (11.43, 49.53) ccw
  arc A4237 (33.02, 44.5262) -> (33.02, 44.3738) centre (33.02, 44.45) ccw
  arc A4238 (60.9061, 45.6661) -> (61.0139, 45.7739) centre (60.96, 45.72) ccw
  line L1463 (40.64, 41.91) -> (43.18, 44.45)
  arc A4239 (39.3161, 44.5039) -> (39.4239, 44.3961) centre (39.37, 44.45) ccw
  line L1464 (60.96, 45.72) -> (59.69, 46.99)
  arc A4240 (69.0047, 10.2139) -> (68.897, 10.1061) centre (68.9509, 10.16) ccw
  line L1465 (58.42, 16.51) -> (67.31, 16.51)
  line L1466 (11.43, 45.72) -> (11.43, 49.53)
  arc A4241 (61.0362, 45.72) -> (60.8838, 45.72) centre (60.96, 45.72) ccw
  arc A4242 (82.7532, 12.446) -> (82.6008, 12.446) centre (82.677, 12.446) ccw
  arc A4243 (82.7309, 9.2781) -> (82.6231, 9.3858) centre (82.677, 9.332) ccw
  arc A4244 (71.6529, 7.3502) -> (71.7606, 7.458) centre (71.7067, 7.4041) ccw
  line L1467 (55.88, 34.29) -> (55.88, 19.05)
  arc A4245 (58.42, 16.5862) -> (58.42, 16.4338) centre (58.42, 16.51) ccw
  line L1468 (43.18, 48.26) -> (44.45, 46.99)
  line L1469 (59.69, 46.99) -> (44.45, 46.99)
  arc A4246 (8.128, 44.5262) -> (8.128, 44.3738) centre (8.128, 44.45) ccw
  arc A4247 (36.7761, 38.1539) -> (36.8839, 38.0461) centre (36.83, 38.1) ccw
  arc A4248 (11.4839, 45.6661) -> (11.3761, 45.7739) centre (11.43, 45.72) ccw
  arc A4249 (30.4261, 41.9639) -> (30.5339, 41.8561) centre (30.48, 41.91) ccw
  line L1470 (60.96, 43.18) -> (60.96, 45.72)
  line L1471 (10.16, 44.45) -> (11.43, 45.72)
  arc A4250 (55.9562, 34.29) -> (55.8038, 34.29) centre (55.88, 34.29) ccw
  arc A4251 (71.7067, 7.4803) -> (71.7067, 7.3279) centre (71.7067, 7.4041) ccw
  arc A4252 (34.29, 38.1762) -> (34.29, 38.0238) centre (34.29, 38.1) ccw
  line L1472 (39.37, 44.45) -> (33.02, 44.45)
  arc A4253 (59.7439, 47.0439) -> (59.6361, 46.9361) centre (59.69, 46.99) ccw
  arc A4254 (43.18, 44.5262) -> (43.18, 44.3738) centre (43.18, 44.45) ccw
  arc A4255 (43.2339, 48.3139) -> (43.1261, 48.2061) centre (43.18, 48.26) ccw
  line L1473 (43.18, 48.26) -> (39.37, 44.45)
  line L1474 (30.48, 35.56) -> (31.75, 34.29)
  arc A4256 (53.34, 44.3738) -> (53.34, 44.5262) centre (53.34, 44.45) ccw
  arc A4257 (40.6939, 41.8561) -> (40.5861, 41.9639) centre (40.64, 41.91) ccw
  arc A4258 (59.69, 46.9138) -> (59.69, 47.0662) centre (59.69, 46.99) ccw
  line L1475 (55.88, 19.05) -> (58.42, 16.51)
  arc A4259 (40.5861, 41.9639) -> (40.6939, 41.8561) centre (40.64, 41.91) ccw
  line L1476 (31.75, 34.29) -> (34.29, 34.29)
  arc A4260 (82.6008, 9.332) -> (82.7532, 9.332) centre (82.677, 9.332) ccw
  line L1477 (71.7067, 7.4041) -> (74.2467, 7.4041)
  arc A4261 (74.2467, 7.3279) -> (74.2467, 7.4803) centre (74.2467, 7.4041) ccw
  line L1478 (82.677, 9.332) -> (82.677, 12.446)
  arc A4262 (43.2562, 49.53) -> (43.1038, 49.53) centre (43.18, 49.53) ccw
  line L1479 (33.02, 44.45) -> (30.48, 41.91)
  line L1480 (36.83, 38.1) -> (40.64, 41.91)
  line L1481 (8.128, 44.45) -> (10.16, 44.45)
  arc A4263 (43.2339, 48.2061) -> (43.1261, 48.3139) centre (43.18, 48.26) ccw
  line L1482 (80.7491, 7.4041) -> (74.2467, 7.4041)
  arc A4264 (60.8838, 43.18) -> (61.0362, 43.18) centre (60.96, 43.18) ccw
  arc A4265 (44.3961, 46.9361) -> (44.5039, 47.0439) centre (44.45, 46.99) ccw
  arc A4266 (33.0739, 44.3961) -> (32.9661, 44.5039) centre (33.02, 44.45) ccw
  arc A4267 (10.16, 44.3738) -> (10.16, 44.5262) centre (10.16, 44.45) ccw
  line L1483 (67.31, 10.16) -> (68.9508, 10.16)
  arc A4268 (67.31, 16.4338) -> (67.31, 16.5862) centre (67.31, 16.51) ccw
  arc A4269 (80.7491, 7.3279) -> (80.7491, 7.4803) centre (80.7491, 7.4041) ccw
  line L1484 (43.18, 49.53) -> (43.18, 48.26)
  arc A4270 (43.1038, 48.26) -> (43.2562, 48.26) centre (43.18, 48.26) ccw
  arc A4271 (43.2339, 44.3961) -> (43.1261, 44.5039) centre (43.18, 44.45) ccw
  arc A4272 (30.5339, 35.6139) -> (30.4261, 35.5061) centre (30.48, 35.56) ccw
  arc A4273 (68.9508, 10.0838) -> (68.9508, 10.2362) centre (68.9508, 10.16) ccw
  arc A4274 (58.3661, 16.4561) -> (58.4739, 16.5639) centre (58.42, 16.51) ccw
  arc A4275 (67.31, 10.2362) -> (67.31, 10.0838) centre (67.31, 10.16) ccw
  arc A4276 (34.29, 34.2138) -> (34.29, 34.3662) centre (34.29, 34.29) ccw
  line L1485 (35.56, 46.99) -> (34.29, 45.72)
  line L1486 (34.29, 38.1) -> (36.83, 38.1)
  arc A4277 (77.2956, 53.9596) -> (77.5596, 53.7832) centre (77.4276, 53.8714) ccw
  arc A4278 (44.45, 47.0662) -> (44.45, 46.9138) centre (44.45, 46.99) ccw
  line L1487 (43.18, 44.45) -> (53.34, 44.45)
  arc A4279 (31.6961, 34.2361) -> (31.8039, 34.3439) centre (31.75, 34.29) ccw
  line L1488 (30.48, 41.91) -> (30.48, 35.56)
  arc A4280 (45.72, 25.4762) -> (45.72, 25.3238) centre (45.72, 25.4) ccw
  arc A4281 (46.2739, 21.7523) -> (46.2739, 22.0698) centre (46.2739, 21.9111) ccw
  arc A4282 (24.765, 45.7962) -> (24.765, 45.6438) centre (24.765, 45.72) ccw
  line L1489 (40.64, 6.35) -> (39.1287, 6.35)
  arc A4283 (35.6139, 46.9361) -> (35.5061, 47.0439) centre (35.56, 46.99) ccw
  arc A4284 (7.6739, 29.2639) -> (7.5661, 29.1561) centre (7.62, 29.21) ccw
  line L1490 (34.29, 45.72) -> (24.765, 45.72)
  arc A4285 (48.26, 25.3238) -> (48.26, 25.4762) centre (48.26, 25.4) ccw
  arc A4286 (29.4513, 49.6888) -> (29.4513, 49.3713) centre (29.4513, 49.5301) ccw
  arc A4287 (39.1287, 6.5087) -> (39.1287, 6.1912) centre (39.1287, 6.35) ccw
  arc A4288 (24.8189, 29.1561) -> (24.7111, 29.2639) centre (24.765, 29.21) ccw
  arc A4289 (35.4838, 46.99) -> (35.6362, 46.99) centre (35.56, 46.99) ccw
  line L1491 (45.72, 25.4) -> (40.64, 30.48)
  arc A4290 (38.1, 6.5088) -> (38.1, 6.1913) centre (38.1, 6.3501) ccw
  arc A4291 (30.3212, 49.53) -> (30.6387, 49.53) centre (30.48, 49.53) ccw
  arc A4292 (39.37, 44.3738) -> (39.37, 44.5262) centre (39.37, 44.45) ccw
  arc A4293 (40.6939, 30.5339) -> (40.5861, 30.4261) centre (40.64, 30.48) ccw
  line L1492 (29.4513, 49.53) -> (30.48, 49.53)
  arc A4294 (30.48, 49.3713) -> (30.48, 49.6888) centre (30.48, 49.5301) ccw
  arc A4295 (38.1, 6.5087) -> (38.1, 6.1912) centre (38.1, 6.35) ccw
  arc A4296 (40.7987, 6.35) -> (40.4812, 6.35) centre (40.6399, 6.35) ccw
  arc A4297 (53.34, 19.3992) -> (53.34, 19.0817) centre (53.34, 19.2405) ccw
  arc A4298 (39.1287, 6.1912) -> (39.1287, 6.5087) centre (39.1287, 6.35) ccw
  arc A4299 (54.6882, 18.2727) -> (54.9128, 18.4972) centre (54.8005, 18.385) ccw
  arc A4300 (40.64, 6.1912) -> (40.64, 6.5087) centre (40.64, 6.35) ccw
  arc A4301 (8.8361, 27.8861) -> (8.9439, 27.9939) centre (8.89, 27.94) ccw
  line L1493 (23.495, 27.94) -> (24.765, 29.21)
  arc A4302 (45.6661, 25.3461) -> (45.7739, 25.4539) centre (45.72, 25.4) ccw
  line L1494 (48.26, 25.4) -> (45.72, 25.4)
  arc A4303 (34.29, 45.6438) -> (34.29, 45.7962) centre (34.29, 45.72) ccw
  arc A4304 (31.75, 34.3662) -> (31.75, 34.2138) centre (31.75, 34.29) ccw
  arc A4305 (40.4812, 6.35) -> (40.7987, 6.35) centre (40.6399, 6.35) ccw
  line L1495 (38.1, 6.35) -> (40.64, 6.35)
  arc A4306 (34.2361, 45.7739) -> (34.3439, 45.6661) centre (34.29, 45.72) ccw
  line L1496 (30.48, 49.53) -> (27.94, 49.53)
  arc A4307 (23.4411, 27.9939) -> (23.5489, 27.8861) centre (23.495, 27.94) ccw
  arc A4308 (76.9116, 52.4192) -> (76.9116, 52.1017) centre (76.9116, 52.2604) ccw
  line L1497 (76.9346, 51.3926) -> (77.0064, 51.0316)
  line L1498 (39.1287, 6.35) -> (38.1, 6.35)
  arc A4309 (8.89, 28.0162) -> (8.89, 27.8638) centre (8.89, 27.94) ccw
  arc A4310 (37.9413, 6.35) -> (38.2588, 6.35) centre (38.1, 6.35) ccw
  line L1499 (7.62, 29.21) -> (8.89, 27.94)
  arc A4311 (30.4038, 35.56) -> (30.5562, 35.56) centre (30.48, 35.56) ccw
  arc A4312 (30.5562, 41.91) -> (30.4038, 41.91) centre (30.48, 41.91) ccw
  arc A4313 (35.6362, 49.53) -> (35.4838, 49.53) centre (35.56, 49.53) ccw
  line L1500 (23.495, 27.94) -> (8.89, 27.94)
  arc A4314 (23.495, 27.8638) -> (23.495, 28.0162) centre (23.495, 27.94) ccw
  line L1501 (35.56, 46.99) -> (35.56, 49.53)
  arc A4315 (38.2588, 6.35) -> (37.9413, 6.35) centre (38.1, 6.35) ccw
  line L1502 (80.3275, 52.2605) -> (80.3275, 51.6255)
  line L1503 (77.8657, 54.462) -> (77.6322, 54.1775)
  arc A4316 (36.83, 38.0238) -> (36.83, 38.1762) centre (36.83, 38.1) ccw
  arc A4317 (40.64, 6.1913) -> (40.64, 6.5088) centre (40.64, 6.3501) ccw
  arc A4318 (30.6387, 49.53) -> (30.3212, 49.53) centre (30.48, 49.53) ccw
  arc A4319 (79.5941, 55.3734) -> (79.5019, 55.6772) centre (79.548, 55.5253) ccw
  arc A4320 (78.2382, 54.6101) -> (78.0137, 54.8346) centre (78.126, 54.7224) ccw
  line L1504 (77.0064, 51.0316) -> (77.1133, 50.6793)
  arc A4321 (76.9613, 50.6332) -> (77.2652, 50.7254) centre (77.1133, 50.6793) ccw
  line L1505 (76.9116, 52.2605) -> (80.3275, 52.2605)
  arc A4322 (77.1621, 52.8235) -> (76.8507, 52.8854) centre (77.0064, 52.8545) ccw
  arc A4323 (27.94, 49.6888) -> (27.94, 49.3713) centre (27.94, 49.5301) ccw
  arc A4324 (79.4421, 55.3281) -> (79.3206, 55.6214) centre (79.3813, 55.4748) ccw
  line L1506 (77.6322, 54.1775) -> (77.4276, 53.8714)
  arc A4325 (78.8048, 55.0284) -> (78.6284, 55.2923) centre (78.7166, 55.1604) ccw
  arc A4326 (77.1583, 51.0777) -> (76.8545, 50.9855) centre (77.0064, 51.0316) ccw
  arc A4327 (79.1161, 55.1939) -> (78.9664, 55.4739) centre (79.0413, 55.3339) ccw
  arc A4328 (77.0926, 52.4778) -> (76.7766, 52.5089) centre (76.9346, 52.4934) ccw
  line L1507 (78.4105, 54.9558) -> (78.126, 54.7223)
  line L1508 (79.0412, 55.3339) -> (78.7166, 55.1604)
  line L1509 (79.3813, 55.4747) -> (79.0412, 55.3339)
  arc A4329 (79.3352, 55.6267) -> (79.4274, 55.3228) centre (79.3813, 55.4747) ccw
  line L1510 (78.126, 54.7223) -> (77.8657, 54.462)
  arc A4330 (76.8507, 51.0006) -> (77.1621, 51.0625) centre (77.0064, 51.0316) ccw
  arc A4331 (77.0903, 51.4236) -> (76.7789, 51.3616) centre (76.9346, 51.3926) ccw
  arc A4332 (78.9805, 55.4805) -> (79.102, 55.1872) centre (79.0413, 55.3338) ccw
  arc A4333 (27.94, 49.6887) -> (27.94, 49.3712) centre (27.94, 49.53) ccw
  arc A4334 (78.6418, 55.3004) -> (78.7914, 55.0203) centre (78.7166, 55.1604) ccw
  arc A4335 (82.1739, 48.6921) -> (82.3236, 48.4121) centre (82.2488, 48.5521) ccw
  arc A4336 (80.4862, 51.6255) -> (80.1688, 51.6255) centre (80.3275, 51.6255) ccw
  arc A4337 (77.0696, 51.6411) -> (76.7537, 51.6099) centre (76.9116, 51.6255) ccw
  line L1511 (77.1133, 53.2067) -> (77.0064, 52.8544)
  arc A4338 (77.5676, 53.7966) -> (77.2876, 53.9462) centre (77.4276, 53.8714) ccw
  arc A4339 (77.9884, 54.3613) -> (77.743, 54.5627) centre (77.8657, 54.462) ccw
  line L1512 (76.9346, 52.4934) -> (76.9116, 52.2605)
  arc A4340 (82.3095, 48.4055) -> (82.188, 48.6988) centre (82.2487, 48.5522) ccw
  line L1513 (78.7166, 55.1604) -> (78.4105, 54.9558)
  arc A4341 (80.3275, 52.1017) -> (80.3275, 52.4192) centre (80.3275, 52.2604) ccw
  arc A4342 (76.7766, 51.377) -> (77.0926, 51.4082) centre (76.9346, 51.3926) ccw
  arc A4343 (77.1141, 53.6216) -> (77.3941, 53.4719) centre (77.2541, 53.5468) ccw
  arc A4344 (78.3223, 55.0878) -> (78.4987, 54.8238) centre (78.4105, 54.9558) ccw
  arc A4345 (80.1687, 51.6255) -> (80.4862, 51.6255) centre (80.3274, 51.6255) ccw
  arc A4346 (28.0988, 49.53) -> (27.7813, 49.53) centre (27.9401, 49.53) ccw
  line L1514 (77.2541, 53.5468) -> (77.1133, 53.2067)
  arc A4347 (77.7641, 54.0893) -> (77.5002, 54.2657) centre (77.6322, 54.1775) ccw
  arc A4348 (78.5112, 54.8331) -> (78.3098, 55.0786) centre (78.4105, 54.9558) ccw
  arc A4349 (76.8545, 52.9005) -> (77.1583, 52.8083) centre (77.0064, 52.8544) ccw
  arc A4350 (77.2652, 53.1606) -> (76.9613, 53.2528) centre (77.1132, 53.2067) ccw
  line L1515 (76.9116, 51.6255) -> (76.9346, 51.3926)
  line L1516 (79.548, 55.5253) -> (79.3813, 55.4747)
  arc A4351 (76.9116, 51.7843) -> (76.9116, 51.4668) centre (76.9116, 51.6256) ccw
  arc A4352 (78.0253, 54.845) -> (78.2267, 54.5996) centre (78.126, 54.7223) ccw
  arc A4353 (76.7537, 52.2761) -> (77.0696, 52.2449) centre (76.9116, 52.2605) ccw
  arc A4354 (80.3275, 51.4668) -> (80.3275, 51.7843) centre (80.3275, 51.6256) ccw
  arc A4355 (77.4008, 53.486) -> (77.1075, 53.6075) centre (77.2542, 53.5468) ccw
  arc A4356 (77.7534, 54.5743) -> (77.9779, 54.3498) centre (77.8657, 54.4621) ccw
  arc A4357 (30.48, 49.3712) -> (30.48, 49.6887) centre (30.48, 49.53) ccw
  arc A4358 (29.4513, 49.3713) -> (29.4513, 49.6888) centre (29.4513, 49.5301) ccw
  arc A4359 (76.9666, 53.2674) -> (77.2599, 53.1459) centre (77.1132, 53.2066) ccw
  arc A4360 (76.7789, 52.5244) -> (77.0903, 52.4624) centre (76.9346, 52.4934) ccw
  line L1517 (77.4276, 53.8714) -> (77.2541, 53.5468)
  arc A4361 (27.7813, 49.53) -> (28.0988, 49.53) centre (27.9401, 49.53) ccw
  arc A4362 (80.4862, 52.2605) -> (80.1687, 52.2605) centre (80.3274, 52.2605) ccw
  line L1518 (77.0064, 52.8544) -> (76.9346, 52.4934)
  line L1519 (80.3275, 51.6255) -> (76.9116, 51.6255)
  arc A4363 (77.5094, 54.2782) -> (77.7549, 54.0768) centre (77.6322, 54.1775) ccw
  line L1520 (27.94, 49.53) -> (29.4513, 49.53)
  line L1521 (78.126, 49.1637) -> (78.4105, 48.9302)
  arc A4364 (79.102, 48.6988) -> (78.9805, 48.4055) centre (79.0413, 48.5522) ccw
  arc A4365 (80.1688, 48.2096) -> (80.4862, 48.2096) centre (80.3275, 48.2096) ccw
  line L1522 (80.9625, 51.6255) -> (80.9625, 48.2096)
  arc A4366 (78.9664, 48.4121) -> (79.1161, 48.6921) centre (79.0413, 48.5521) ccw
  arc A4367 (77.5002, 49.6203) -> (77.7641, 49.7967) centre (77.6322, 49.7085) ccw
  arc A4368 (80.9469, 48.3676) -> (80.9781, 48.0517) centre (80.9625, 48.2097) ccw
  line L1523 (77.4276, 50.0146) -> (77.6322, 49.7085)
  arc A4369 (80.1102, 48.3906) -> (80.079, 48.0746) centre (80.0946, 48.2326) ccw
  arc A4370 (78.2267, 49.2864) -> (78.0253, 49.041) centre (78.126, 49.1637) ccw
  arc A4371 (81.2109, 48.0746) -> (81.1798, 48.3906) centre (81.1954, 48.2326) ccw
  arc A4372 (82.4852, 48.8576) -> (82.6616, 48.5936) centre (82.5734, 48.7256) ccw
  line L1524 (80.9625, 48.2096) -> (81.1954, 48.2326)
  line L1525 (81.9087, 48.4113) -> (82.2488, 48.5521)
  arc A4373 (77.2599, 50.7401) -> (76.9666, 50.6186) centre (77.1133, 50.6793) ccw
  line L1526 (77.6322, 49.7085) -> (77.8657, 49.424)
  line L1527 (77.2541, 50.3392) -> (77.4276, 50.0146)
  arc A4374 (77.743, 49.3233) -> (77.9884, 49.5247) centre (77.8657, 49.424) ccw
  arc A4375 (81.5874, 48.1487) -> (81.5255, 48.4601) centre (81.5564, 48.3044) ccw
  line L1528 (77.1133, 50.6793) -> (77.2541, 50.3392)
  arc A4376 (78.6284, 48.5936) -> (78.8048, 48.8576) centre (78.7166, 48.7256) ccw
  arc A4377 (78.3098, 48.8074) -> (78.5112, 49.0529) centre (78.4105, 48.9301) ccw
  arc A4378 (79.6875, 48.1525) -> (79.7797, 48.4563) centre (79.7336, 48.3044) ccw
  arc A4379 (79.7645, 48.4601) -> (79.7026, 48.1487) centre (79.7335, 48.3044) ccw
  arc A4380 (81.1212, 51.6255) -> (80.8037, 51.6255) centre (80.9624, 51.6255) ccw
  arc A4381 (80.0636, 48.0769) -> (80.1256, 48.3883) centre (80.0946, 48.2326) ccw
  arc A4382 (78.7914, 48.8656) -> (78.6418, 48.5856) centre (78.7166, 48.7256) ccw
  arc A4383 (81.1644, 48.3883) -> (81.2264, 48.0769) centre (81.1954, 48.2326) ccw
  line L1529 (79.3813, 48.4113) -> (79.7336, 48.3044)
  arc A4384 (78.0137, 49.0514) -> (78.2382, 49.2759) centre (78.126, 49.1637) ccw
  line L1530 (80.3275, 51.6255) -> (80.9625, 51.6255)
  line L1531 (78.7166, 48.7256) -> (79.0412, 48.5521)
  arc A4385 (78.4987, 49.0621) -> (78.3223, 48.7982) centre (78.4105, 48.9302) ccw
  arc A4386 (82.6482, 48.5856) -> (82.4986, 48.8656) centre (82.5734, 48.7256) ccw
  line L1532 (81.1954, 48.2326) -> (81.5564, 48.3044)
  arc A4387 (77.9779, 49.5362) -> (77.7534, 49.3117) centre (77.8657, 49.424) ccw
  arc A4388 (81.5103, 48.4563) -> (81.6025, 48.1525) centre (81.5564, 48.3044) ccw
  arc A4389 (80.8037, 48.2096) -> (81.1212, 48.2096) centre (80.9624, 48.2096) ccw
  arc A4390 (77.3941, 50.4141) -> (77.1141, 50.2644) centre (77.2541, 50.3392) ccw
  arc A4391 (80.9625, 51.4667) -> (80.9625, 51.7842) centre (80.9625, 51.6255) ccw
  line L1533 (77.8657, 49.424) -> (78.126, 49.1637)
  line L1534 (79.0412, 48.5521) -> (79.3813, 48.4113)
  line L1535 (79.7336, 48.3044) -> (80.0946, 48.2326)
  arc A4392 (82.9677, 48.7982) -> (82.7913, 49.0621) centre (82.8795, 48.9301) ccw
  arc A4393 (81.8479, 48.5579) -> (81.9694, 48.2646) centre (81.9086, 48.4113) ccw
  line L1536 (82.2488, 48.5521) -> (82.5734, 48.7256)
  line L1537 (81.5564, 48.3044) -> (81.9087, 48.4113)
  line L1538 (82.8795, 48.9302) -> (83.164, 49.1637)
  line L1539 (82.5734, 48.7256) -> (82.8795, 48.9302)
  line L1540 (78.4105, 48.9302) -> (78.7166, 48.7256)
  arc A4394 (77.1075, 50.2785) -> (77.4008, 50.4) centre (77.2542, 50.3392) ccw
  arc A4395 (77.7549, 49.8092) -> (77.5094, 49.6078) centre (77.6321, 49.7085) ccw
  arc A4396 (77.5596, 50.1028) -> (77.2956, 49.9264) centre (77.4276, 50.0146) ccw
  arc A4397 (79.4274, 48.5632) -> (79.3352, 48.2593) centre (79.3813, 48.4113) ccw
  arc A4398 (81.9548, 48.2593) -> (81.8626, 48.5632) centre (81.9087, 48.4113) ccw
  arc A4399 (79.3206, 48.2646) -> (79.4421, 48.5579) centre (79.3813, 48.4113) ccw
  arc A4400 (77.2876, 49.9398) -> (77.5676, 50.0894) centre (77.4276, 50.0146) ccw
  line L1541 (80.0946, 48.2326) -> (80.3275, 48.2096)
  line L1542 (80.3275, 48.2096) -> (80.3275, 51.6255)
  arc A4401 (80.3275, 51.7842) -> (80.3275, 51.4667) centre (80.3275, 51.6255) ccw
  arc A4402 (80.3119, 48.0517) -> (80.3431, 48.3676) centre (80.3275, 48.2097) ccw
  arc A4403 (84.0248, 50.7254) -> (84.3287, 50.6332) centre (84.1767, 50.6793) ccw
  line L1543 (68.5509, 3.4741) -> (68.5351, 3.5536)
  line L1544 (83.6578, 49.7085) -> (83.8624, 50.0146)
  arc A4404 (68.4001, 1.0601) -> (68.7176, 1.0601) centre (68.5589, 1.0601) ccw
  arc A4405 (68.5292, 3.9333) -> (68.2652, 3.7569) centre (68.3972, 3.8451) ccw
  arc A4406 (68.3831, 3.5075) -> (68.687, 3.5997) centre (68.535, 3.5536) ccw
  line L1545 (68.5115, 3.6312) -> (68.4805, 3.7062)
  arc A4407 (68.2745, 3.7444) -> (68.5199, 3.9458) centre (68.3972, 3.8451) ccw
  line L1546 (83.164, 49.1637) -> (83.4243, 49.424)
  line L1547 (68.3457, 3.9078) -> (68.2884, 3.9652)
  arc A4408 (83.5258, 49.7967) -> (83.7898, 49.6203) centre (83.6578, 49.7085) ccw
  line L1548 (84.2253, 0.7747) -> (68.4918, 0.7747)
  line L1549 (68.5115, 0.8222) -> (68.5351, 0.8998)
  arc A4409 (68.7066, 0.9484) -> (68.3952, 1.0104) centre (68.5509, 0.9794) ccw
  arc A4410 (84.1759, 50.2644) -> (83.8959, 50.4141) centre (84.0359, 50.3392) ccw
  arc A4411 (68.4918, 0.9334) -> (68.4918, 0.6159) centre (68.4918, 0.7747) ccw
  arc A4412 (84.3772, 50.7933) -> (84.0734, 50.8855) centre (84.2253, 50.8394) ccw
  arc A4413 (68.5822, 3.8525) -> (68.3022, 3.7029) centre (68.4422, 3.7777) ccw
  arc A4414 (68.3405, 3.6313) -> (68.6205, 3.781) centre (68.4805, 3.7062) ccw
  arc A4415 (68.7176, 3.3934) -> (68.4001, 3.3934) centre (68.5589, 3.3934) ccw
  arc A4416 (84.2253, 0.6159) -> (84.2253, 0.9334) centre (84.2253, 0.7747) ccw
  arc A4417 (68.3952, 3.4431) -> (68.7066, 3.505) centre (68.5509, 3.474) ccw
  arc A4418 (84.3234, 50.6186) -> (84.0301, 50.7401) centre (84.1767, 50.6794) ccw
  arc A4419 (83.0518, 49.2759) -> (83.2763, 49.0514) centre (83.1641, 49.1637) ccw
  line L1550 (68.5588, 1.0601) -> (68.5588, 3.3934)
  arc A4420 (83.7223, 50.0894) -> (84.0024, 49.9398) centre (83.8624, 50.0146) ccw
  arc A4421 (68.7089, 3.4896) -> (68.3929, 3.4585) centre (68.5509, 3.474) ccw
  line L1551 (68.5351, 0.8998) -> (68.5509, 0.9794)
  arc A4422 (84.0666, 0.7747) -> (84.3841, 0.7747) centre (84.2253, 0.7747) ccw
  arc A4423 (68.4684, 4.0085) -> (68.223, 3.8071) centre (68.3457, 3.9078) ccw
  line L1552 (83.4243, 49.424) -> (83.6578, 49.7085)
  line L1553 (68.3972, 3.8451) -> (68.3457, 3.9078)
  arc A4424 (68.3452, 0.8355) -> (68.6385, 0.7139) centre (68.4919, 0.7747) ccw
  line L1554 (84.0359, 50.3392) -> (84.1767, 50.6793)
  arc A4425 (68.7168, 1.0446) -> (68.4008, 1.0757) centre (68.5588, 1.0601) ccw
  arc A4426 (83.9943, 49.9264) -> (83.7304, 50.1028) centre (83.8624, 50.0146) ccw
  arc A4427 (68.6634, 3.6773) -> (68.3596, 3.5852) centre (68.5115, 3.6312) ccw
  line L1555 (68.4918, 0.7747) -> (68.5115, 0.8222)
  arc A4428 (68.3596, 0.8683) -> (68.6634, 0.7761) centre (68.5115, 0.8222) ccw
  arc A4429 (68.6271, 3.7669) -> (68.3338, 3.6454) centre (68.4805, 3.7062) ccw
  arc A4430 (68.3929, 0.995) -> (68.7089, 0.9638) centre (68.5509, 0.9794) ccw
  arc A4431 (68.3794, 0.9308) -> (68.6908, 0.8689) centre (68.5351, 0.8999) ccw
  line L1556 (68.5588, 3.3934) -> (68.5509, 3.4741)
  line L1557 (68.4805, 3.7062) -> (68.4422, 3.7777)
  arc A4432 (68.4006, 4.0774) -> (68.1761, 3.8529) centre (68.2884, 3.9651) ccw
  line L1558 (68.5509, 0.9794) -> (68.5588, 1.0601)
  line L1559 (68.5351, 3.5536) -> (68.5115, 3.6312)
  arc A4433 (83.8892, 50.4) -> (84.1825, 50.2785) centre (84.0359, 50.3393) ccw
  arc A4434 (83.7806, 49.6078) -> (83.5351, 49.8092) centre (83.6579, 49.7085) ccw
  arc A4435 (68.3102, 3.6895) -> (68.5742, 3.8659) centre (68.4422, 3.7777) ccw
  arc A4436 (68.6908, 3.5846) -> (68.3794, 3.5227) centre (68.5351, 3.5537) ccw
  arc A4437 (82.7788, 49.0529) -> (82.9802, 48.8074) centre (82.8795, 48.9301) ccw
  arc A4438 (84.3841, 50.8394) -> (84.0666, 50.8394) centre (84.2253, 50.8394) ccw
  arc A4439 (83.5366, 49.3117) -> (83.3121, 49.5362) centre (83.4244, 49.424) ccw
  line L1560 (84.2253, 50.8394) -> (84.2253, 0.7747)
  arc A4440 (68.4008, 3.3778) -> (68.7168, 3.4089) centre (68.5588, 3.3934) ccw